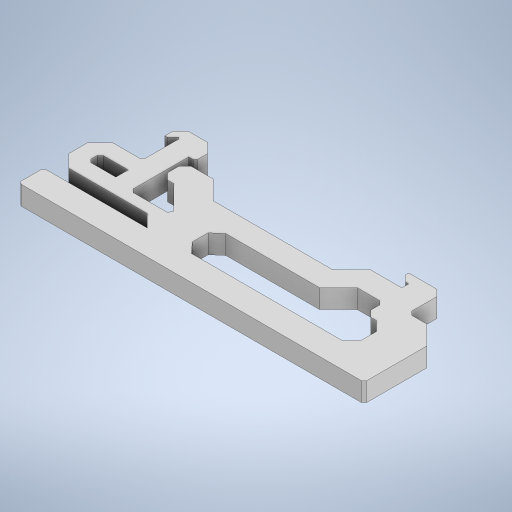
# Autodesk Inventor part: CO_1_01_dinRail
Saved by Autodesk Inventor 2023 (Build 270158000, 158)
## iProperties
Created: 2023-01-23
Part Number: CO_1_01_dinRail
Material: Generic
Document SubType Name: Modeling
Designer: t205b
Density: 1 g/cm^3
Appearance: Default
Author: t205b
Autodesk Inventor part; units mm, degrees
ref_plane "YZ Plane" through (0, 0, 0) normal (1, 0, 0) x (0, 1, 0)
ref_plane "XZ Plane" through (0, 0, 0) normal (0, 1, 0) x (-1, 0, 0)
ref_plane "XY Plane" through (0, 0, 0) normal (0, 0, 1) x (1, 0, 0)
sketch "Sketch1" plane through (0, 0, 0) normal (0, 1, 0) x (-1, 0, 0)
  line L0 (-17.6312, -19.1085) -> (1.2602, -19.1085)
  line L1 (-32.5455, -19.1086) -> (-30.1592, -19.1086)
  line L2 (-33.9375, -17.7166) -> (-32.5455, -19.1086)
  line L3 (-35.5284, -16.1257) -> (-33.9375, -17.7166)
  line L4 (2.9824, -14.5915) -> (3.2737, -13.8887)
  line L5 (-2.717, -14.3021) -> (-4.2084, -15.6146)
  line L6 (-2.717, -11.8304) -> (-4.2084, -10.16)
  line L7 (18.7576, -6.1828) -> (-35.133, -6.1828)
  line L8 (18.7597, -10.1584) -> (2.7517, -10.1584)
  line L9 (-29.5627, -14.1232) -> (-28.0713, -15.6146)
  line L10 (18.7576, -6.1828) -> (19.157, -6.5801)
  line L11 (19.157, -6.5801) -> (19.157, -9.7618)
  line L12 (19.157, -9.7618) -> (18.7597, -10.1584)
  line L13 (2.7517, -10.1584) -> (4.7402, -12.147)
  line L14 (4.7402, -12.147) -> (17.1688, -12.147)
  line L15 (17.1688, -12.147) -> (19.1574, -14.1355)
  line L16 (19.1574, -14.1355) -> (19.1574, -17.1184)
  line L17 (19.1574, -17.1184) -> (17.1688, -19.107)
  line L18 (17.1688, -19.107) -> (12.9431, -19.107)
  line L19 (12.9431, -19.107) -> (12.4459, -19.6041)
  line L20 (12.4459, -19.6041) -> (12.4459, -24.8441)
  line L21 (12.4459, -24.8441) -> (12.6845, -25.0822)
  line L22 (12.6845, -25.0822) -> (13.5894, -24.1758)
  line L23 (13.5894, -24.1758) -> (13.9871, -24.1758)
  line L24 (13.9871, -24.1758) -> (13.9871, -25.4685)
  line L25 (13.9871, -25.4685) -> (12.7939, -26.6636)
  line L26 (12.7939, -26.6636) -> (9.7117, -26.6636)
  line L27 (9.7117, -26.6636) -> (8.1705, -25.1225)
  line L28 (8.1705, -23.5316) -> (8.1705, -25.1225)
  line L29 (8.5185, -23.1836) -> (9.2145, -23.1836)
  line L30 (2.9824, -14.5915) -> (6.7288, -18.3379)
  line L31 (6.7288, -18.3379) -> (7.7231, -18.3379)
  line L32 (7.7231, -18.3379) -> (8.7174, -19.3322)
  line L33 (8.7174, -19.3322) -> (8.7174, -21.097)
  line L34 (8.7174, -21.097) -> (7.7231, -22.0913)
  line L35 (7.7231, -22.0913) -> (4.2431, -22.0913)
  line L36 (4.2431, -22.0913) -> (1.2602, -19.1085)
  line L37 (-17.6312, -19.1085) -> (-20.6141, -22.0913)
  line L38 (-20.6141, -22.0913) -> (-25.5855, -22.0913)
  line L39 (-25.5855, -22.0913) -> (-25.5855, -23.1851)
  line L40 (-25.5855, -23.1851) -> (-25.0884, -23.1851)
  line L41 (-25.0884, -23.1851) -> (-24.0941, -24.1794)
  line L42 (-24.0941, -24.1794) -> (-24.0941, -24.6766)
  line L43 (-24.0941, -24.6766) -> (-28.5683, -24.6766)
  line L44 (-28.5683, -24.6766) -> (-29.5626, -23.6823)
  line L45 (-29.5626, -23.6823) -> (-29.5626, -19.7051)
  line L46 (-29.5626, -19.7051) -> (-30.1592, -19.1086)
  line L47 (-35.5284, -16.1257) -> (-35.5284, -6.5807)
  line L48 (-35.5284, -6.5807) -> (-35.133, -6.1828)
  line L49 (-29.5627, -14.1232) -> (-29.5627, -11.6514)
  line L50 (-29.5627, -11.6514) -> (-28.0713, -10.16)
  line L51 (-28.0713, -10.16) -> (-4.2084, -10.16)
  line L52 (-2.717, -11.8304) -> (-2.717, -14.3021)
  line L53 (-4.2084, -15.6146) -> (-19.0784, -15.6146)
  line L54 (-22.0613, -18.5974) -> (-25.5855, -18.5974)
  line L55 (-26.1821, -16.6089) -> (-27.1764, -15.6146)
  line L56 (-26.1821, -18.0009) -> (-26.1821, -16.6089)
  line L57 (-27.1764, -15.6146) -> (-28.0713, -15.6146)
  line L58 (-25.5855, -18.5974) -> (-26.1821, -18.0009)
  line L59 (-19.0784, -15.6146) -> (-22.0613, -18.5974)
  line L60 (12.211, -16.6077) -> (12.211, -14.6465)
  line L61 (12.211, -14.6465) -> (16.1607, -14.6465)
  line L62 (16.1607, -14.6465) -> (16.6579, -15.1437)
  line L63 (16.6579, -15.1437) -> (16.6579, -16.1106)
  line L64 (16.6579, -16.1106) -> (16.1607, -16.6077)
  line L65 (16.1607, -16.6077) -> (12.211, -16.6077)
  line L66 (8.5185, -23.1836) -> (8.1705, -23.5316)
  line L67 (9.2145, -14.3859) -> (9.2145, -23.1836)
  line L68 (8.7174, -13.8887) -> (9.2145, -14.3859)
  line L69 (8.7174, -13.8887) -> (3.2737, -13.8887)
  point P0 (0, 0)
  point P1 (-29.5627, -12.8873)
  dimension "d2" = 9.545
  dimension "d3" = 3.9771
  dimension "d4" = 4.4743
  dimension "d6" = 4.9714
  dimension "d7" = 3.5242
  dimension "d9" = 2.9829
  dimension "d11" = 0.9943
  dimension "d12" = 0.398
  dimension "d13" = 53.8907
  dimension "d14" = 2.4718
  dimension "d15" = 1.4914
  dimension "d16" = 1.4914
  dimension "d18" = 1.392
  dimension "d19" = 0.5966
  dimension "d20" = 23.8629
  dimension "d21" = 1.4914
  dimension "d22" = 2.4718
  dimension "d23" = 14.8701
  dimension "d24" = 2.9829
  dimension "d25" = 18.8914
  dimension "d27" = 2.9829
  dimension "d28" = 2.9829
  dimension "d29" = 3.48
  dimension "d30" = 3.7464
  dimension "d31" = 0.7028
  dimension "d32" = 5.4437
  dimension "d33" = 8.7978
  dimension "d34" = 0.4971
  dimension "d35" = 1.5909
  dimension "d36" = 0.348
  dimension "d37" = 0.696
  dimension "d38" = 1.5411
  dimension "d39" = 3.0823
  dimension "d40" = 1.1931
  dimension "d41" = 1.2927
  dimension "d42" = 0.3977
  dimension "d43" = 0.9048
  dimension "d44" = 0.2386
  dimension "d45" = 5.24
  dimension "d46" = 0.4971
  dimension "d47" = 4.2257
  dimension "d48" = 1.9886
  dimension "d49" = 2.9829
  dimension "d50" = 1.9886
  dimension "d51" = 12.4286
  dimension "d52" = 1.9886
  dimension "d54" = 16.008
  dimension "d55" = 0.3973
  dimension "d56" = 3.1817
  dimension "d58" = 2.9829
  dimension "d59" = 2.9829
  dimension "d60" = 2.9829
  dimension "d61" = 0.9943
  dimension "d62" = 0.9943
  dimension "d63" = 0.9943
  dimension "d64" = 3.7463
  dimension "d66" = 1.7649
  dimension "d67" = 0.9943
  dimension "d68" = 0.9943
  dimension "d69" = 0.4971
  dimension "d75" = 0.4971
  dimension "d76" = 0.4971
  dimension "d77" = 0.4971
  dimension "d78" = 0.4971
  constraints: 140 end point, 26 parallel, 17 perpendicular, 3 vertical, 1 horizontal, 1 midpoint
  measures "d2" distance of L47.end L3.start
  measures "d3" distance of L45.end L44.end
  measures "d4" distance of L43.end L42.end
  measures "d6" distance of L38.end L37.end
  measures "d7" distance of L54.start L54.end
  measures "d9" horizontal distance of L1.start L3.start
  measures "d11" horizontal distance of L44.end L43.end
  measures "d12" vertical distance of L7.end L47.end
  measures "d13" distance of L7.start L7.end
  measures "d14" distance of L9.start L49.end
  measures "d15" horizontal distance of L49.end L50.end
  measures "d16" horizontal distance of L9.start L9.end
  measures "d18" distance of L56.start L55.start
  measures "d19" vertical distance of L54.end L56.start
  measures "d20" distance of L50.end L6.end
  measures "d21" horizontal distance of L6.start L6.end
  measures "d22" distance of L6.start L5.start
  measures "d23" distance of L5.end L53.end
  measures "d24" horizontal distance of L53.end L54.start
  measures "d25" distance of L0.end L0.start
  measures "d27" horizontal distance of L37.end L0.start
  measures "d28" horizontal distance of L0.end L35.end
  measures "d29" distance of L35.end L34.end
  measures "d30" horizontal distance of L30.end L4.start
  measures "d31" vertical distance of L4.start L4.end
  measures "d32" distance of L4.end L68.start
  measures "d33" distance of L67.start L29.end
  measures "d34" horizontal distance of L68.start L67.start
  measures "d35" distance of L28.start L27.end
  measures "d36" horizontal distance of L28.start L29.start
  measures "d37" distance of L29.end L29.start
  measures "d38" horizontal distance of L27.end L26.end
  measures "d39" distance of L26.end L25.end
  measures "d40" horizontal distance of L25.end L24.end
  measures "d41" distance of L24.end L23.end
  measures "d42" distance of L23.end L22.end
  measures "d43" horizontal distance of L22.end L21.end
  measures "d44" horizontal distance of L21.end L20.end
  measures "d45" distance of L20.end L19.end
  measures "d46" horizontal distance of L19.end L18.end
  measures "d47" distance of L18.end L17.end
  measures "d48" horizontal distance of L16.end L17.end
  measures "d49" distance of L15.end L16.end
  measures "d50" horizontal distance of L14.end L15.end
  measures "d51" distance of L14.end L13.end
  measures "d52" horizontal distance of L8.end L13.end
  measures "d54" distance of L8.end L8.start
  measures "d55" horizontal distance of L8.start L11.end
  measures "d56" distance of L11.end L10.end
  measures "d58" horizontal distance of L37.end L0.start
  measures "d59" horizontal distance of L53.end L54.start
  measures "d60" horizontal distance of L0.end L35.end
  measures "d61" horizontal distance of L32.end L31.end
  measures "d62" horizontal distance of L32.end L31.end
  measures "d63" distance of L31.end L30.end
  measures "d64" vertical distance of L30.end L4.start
  measures "d66" distance of L33.end L32.end
  measures "d67" horizontal distance of L34.end L33.end
  measures "d68" horizontal distance of L34.end L33.end
  measures "d69" horizontal distance of L19.end L18.end
  measures "d75" horizontal distance of L63.end L64.end
  measures "d76" horizontal distance of L63.end L64.end
  measures "d77" horizontal distance of L61.end L62.end
  measures "d78" horizontal distance of L61.end L62.end
extrude "Extrusion1" add sketch "Sketch1" along normal blind 3
body "Solid1"
